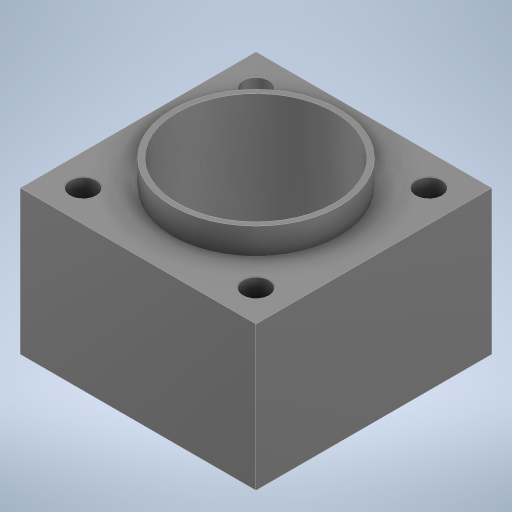
# Autodesk Inventor part: 2309HCMUTE-CDT23-NAP_DUOI
Saved by Autodesk Inventor 2023 (Build 270158000, 158)
## iProperties
Created: 2023-03-30
Part Number: 2309HCMUTE-CDT23-NAP_DUOI
Material: Generic
Document SubType Name: Modeling
Designer: havie
Density: 1 g/cm^3
Appearance: Default
Sending System: SolidWorks 2013
Last Author: win7
Last Saved: 2023-03-30
Author: havie
Autodesk Inventor part; units mm, degrees
ref_plane "YZ Plane" through (0, 0, 0) normal (1, 0, 0) x (0, 1, 0)
ref_plane "XZ Plane" through (0, 0, 0) normal (0, 1, 0) x (-1, 0, 0)
ref_plane "XY Plane" through (0, 0, 0) normal (0, 0, 1) x (1, 0, 0)
sketch "Sketch1" plane through (0, 0, 0) normal (0, 1, 0) x (-1, 0, 0)
  line L0 (22.5, 22.5) -> (-22.5, 22.5)
  line L1 (-22.5, 22.5) -> (-22.5, -22.5)
  line L2 (-22.5, -22.5) -> (22.5, -22.5)
  line L3 (22.5, -22.5) -> (22.5, 22.5)
  line L4 (22.5, 22.5) -> (-22.5, -22.5) construction
  line L5 (-22.5, 22.5) -> (22.5, -22.5) construction
  point P0 (0, 0)
  dimension "d0" = 45
  dimension "d1" = 45
  constraints: 12 end point, 2 midpoint, 2 parallel, 1 horizontal, 1 perpendicular
  measures "d0" distance of L0.end L1.end
  measures "d1" distance of L1.end L2.end
extrude "Extrusion1" add sketch "Sketch1" along normal blind 27.5
sketch "Sketch2" plane through (0, 27.5, 0) normal (0, 1, 0) x (1, 0, 0)
  circle A0 centre (0, 0) radius 16
  dimension "d4" = 32
  constraints: 1 centre point, 1 coincident
  measures "d4" diameter of A0
extrude "Extrusion2" add sketch "Sketch2" along normal blind 5
sketch "Sketch4" plane through (0, 0, 0) normal (0, -1, 0) x (1, 0, 0)
  point P0 (0, 0)
  point P1 (16.5, -16.5)
  point P2 (-16.5, -16.5)
  point P3 (-16.5, 16.5)
  point P4 (16.5, 16.5)
  dimension "d8" = 33
  dimension "d9" = 16.5
  dimension "d10" = 33
  dimension "d11" = 16.5
  constraints: 2 horizontal alignment, 2 vertical alignment
  measures "d8" distance of point (-16.5, -16.5) point (16.5, -16.5)
  measures "d9" horizontal distance of point (0, 0) point (-16.5, -16.5)
  measures "d10" distance of point (-16.5, 16.5) point (-16.5, -16.5)
  measures "d11" horizontal distance of point (0, 0) point (-16.5, 16.5)
hole "Hole1" at (16.5, 0, -16.5) at (-16.5, 0, -16.5) at (-16.5, 0, 16.5) at (16.5, 0, 16.5) direction (0, 1, 0) diameter 4.917 depth 9.5 tip angle 118 thread size "M6x1" class "6H" standard "ISO Metric profile"
sketch "Sketch3" plane through (0, 32.5, 0) normal (0, 1, 0) x (1, 0, 0)
  circle A0 centre (0, 0) radius 15
  dimension "d7" = 30
  constraints: 1 centre point, 1 coincident
  measures "d7" diameter of A0
extrude "Extrusion3" cut sketch "Sketch3" against normal blind 28
sketch "Sketch5" plane through (0, 27.5, 0) normal (0, 1, 0) x (1, 0, 0)
  circle A0 centre (16.5, 16.5) radius 2.4585 projected
  circle A1 centre (16.5, -16.5) radius 2.4585 projected
  circle A2 centre (-16.5, -16.5) radius 2.4585 projected
  circle A3 centre (-16.5, 16.5) radius 2.4585 projected
  point P0 (0, 0)
  constraints: 4 coincident
hole "Hole2" at (16.5, 27.5, -16.5) at (16.5, 27.5, 16.5) at (-16.5, 27.5, 16.5) at (-16.5, 27.5, -16.5) direction (0, -1, 0) diameter 5 depth 10 tip angle 118
sketch "Sketch6" plane through (-22.5, 0, -22.5) normal (-1, 0, 0) x (0, 0, 1)
  line L0 (45, 0) -> (45, 27.5) projected
  line L1 (0, 27.5) -> (45, 27.5) projected
  point P0 (22.5, 0)
  point P1 (25, 12.5)
  dimension "d28" = 20
  dimension "d29" = 15
  measures "d28" distance from line of L0 point (25, 12.5)
  measures "d29" distance from line of L1 point (25, 12.5)
hole "Hole3" at (-22.5, 12.5, 2.5) direction (1, 0, 0) diameter 7.9175 depth 27.5375 tip angle 118 thread size "M9x1" class "6H" standard "ISO Metric profile"
equation "\"d11\" = d9"
body "Solid1"
body "Solid2"
